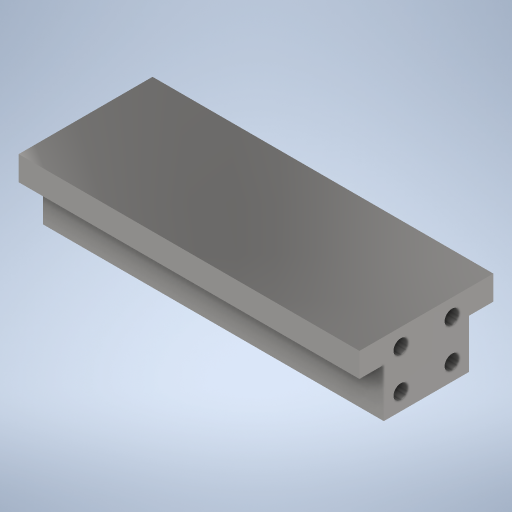
# Autodesk Inventor part: Fuhrung
Saved by Autodesk Inventor 2023.2 (Build 272271000, 271)
## iProperties
Created: 2023-02-02
Part Number: Fuhrung
Material: Steel, Mild
Document SubType Name: Modeling
Designer: Aditya
Density: 7.85 g/cm^3
Appearance: Semi-Polished
Author: Aditya
Autodesk Inventor part; units mm, degrees
ref_plane "YZ Plane" through (0, 0, 0) normal (1, 0, 0) x (0, 1, 0)
ref_plane "XZ Plane" through (0, 0, 0) normal (0, 1, 0) x (-1, 0, 0)
ref_plane "XY Plane" through (0, 0, 0) normal (0, 0, 1) x (1, 0, 0)
sketch "Sketch1" plane through (0, 0, 0) normal (1, 0, 0) x (0, 1, 0)
  line L0 (30, 0) -> (30, -55)
  line L1 (30, -55) -> (20, -55)
  line L2 (20, -55) -> (20, -45)
  line L3 (20, -45) -> (0, -45)
  line L4 (0, -45) -> (0, -10)
  line L5 (0, -10) -> (20, -10)
  line L6 (20, -10) -> (20, 0)
  line L7 (20, 0) -> (30, 0)
  point P0 (0, 0)
  dimension "d0" = 55
  dimension "d1" = 10
  dimension "d2" = 10
  dimension "d3" = 20
  dimension "d4" = 35
  dimension "d5" = 20
  dimension "d6" = 10
  dimension "d7" = 30
  dimension "d8" = 0
  constraints: 16 end point, 4 perpendicular, 2 point on line, 1 vertical
  measures "d0" distance of L0.start L0.end
  measures "d1" distance of L0.end L1.end
  measures "d2" distance of L1.end L2.end
  measures "d3" distance of L2.end L3.end
  measures "d4" distance of L3.end L4.end
  measures "d5" distance of L4.end L5.end
  measures "d6" distance of L5.end L6.end
  measures "d7" distance from line of point (0, 0) L0
  measures "d8" distance from line of point (0, 0) L7
extrude "Extrusion1" add sketch "Sketch1" against normal blind 140
sketch "Sketch3" plane through (0, 0, 0) normal (1, 0, 0) x (0, 0, -1)
  line L0 (55, 30) -> (0, 30) projected
  line L1 (10, 20) -> (10, 0) projected
  line L2 (45, 0) -> (45, 20) projected
  line L3 (10, 0) -> (45, 0) projected
  point P0 (0, 0)
  point P1 (17, 23)
  point P2 (38, 23)
  point P3 (17, 7)
  point P4 (38, 7)
  dimension "d26" = 7
  dimension "d27" = 7
  dimension "d28" = 7
  dimension "d29" = 7
  dimension "d30" = 7
  dimension "d31" = 7
  dimension "d32" = 7
  dimension "d33" = 7
  measures "d26" distance from line of L0 point (17, 23)
  measures "d27" distance from line of L1 point (17, 23)
  measures "d28" distance from line of L0 point (38, 23)
  measures "d29" distance from line of L2 point (38, 23)
  measures "d30" distance from line of L3 point (17, 7)
  measures "d31" distance from line of L3 point (38, 7)
  measures "d32" distance from line of L2 point (38, 7)
  measures "d33" distance from line of L1 point (17, 7)
hole "Hole2" at (0, 23, -17) at (0, 23, -38) at (0, 7, -38) at (0, 7, -17) direction (-1, 0, 0) diameter 4.917 depth 20 tip angle 118 counterbore diameter 6 counterbore depth 15 thread size "M6x1" class "6H" standard "ISO Metric profile"
sketch "Sketch4" plane through (-140, 0, 0) normal (-1, 0, 0) x (0, 0, 1)
  line L0 (-45, 0) -> (-10, 0) projected
  line L1 (-45, 20) -> (-45, 0) projected
  line L2 (-10, 0) -> (-10, 20) projected
  point P0 (0, 0)
  point P1 (-38, 23)
  point P2 (-17, 23)
  point P3 (-27.6865, 8)
  dimension "d41" = 8
  dimension "d42" = 23
  dimension "d43" = 23
  dimension "d44" = 7
  dimension "d45" = 7
  measures "d41" distance from line of L0 point (-27.686, 8)
  measures "d42" distance from line of L0 point (-38, 23)
  measures "d43" distance from line of L0 point (-17, 23)
  measures "d44" distance from line of L1 point (-38, 23)
  measures "d45" distance from line of L2 point (-17, 23)
hole "Hole3" at (-140, 8, -27.6865) at (-140, 23, -38) at (-140, 23, -17) direction (1, 0, 0) diameter 4.917 depth 20 tip angle 118 counterbore diameter 6 counterbore depth 15 thread size "M6x1" class "6H" standard "ISO Metric profile"
sketch "Sketch5" plane through (0, 0, -45) normal (0, -1, 0) x (1, 0, 0)
  line L0 (0, 35) -> (0, 0) projected
  line L1 (0, 45) -> (-140, 45) projected
  line L2 (0, -10) -> (-140, -10) projected
  point P0 (-115, 30)
  point P1 (-70, 30)
  point P2 (-25, 30)
  point P3 (-115, 5)
  point P4 (-70, 5)
  point P5 (-25, 5)
  dimension "d53" = 25
  dimension "d61" = 25
  dimension "d62" = 15
  dimension "d63" = 15
  dimension "d64" = 15
  dimension "d65" = 15
  dimension "d66" = 15
  dimension "d67" = 15
  dimension "d68" = 45
  dimension "d69" = 45
  dimension "d70" = 45
  dimension "d71" = 45
  measures "d53" distance from line of L0 point (-25, 30)
  measures "d61" distance from line of L0 point (-25, 5)
  measures "d62" distance from line of point (-25, 30) L1
  measures "d63" distance from line of L1 point (-70, 30)
  measures "d64" distance from line of L1 point (-115, 30)
  measures "d65" distance from line of L2 point (-25, 5)
  measures "d66" distance from line of L2 point (-70, 5)
  measures "d67" distance from line of L2 point (-115, 5)
  measures "d68" distance of point (-25, 30) point (-70, 30)
  measures "d69" distance of point (-25, 5) point (-70, 5)
  measures "d70" distance of point (-70, 5) point (-115, 5)
  measures "d71" distance of point (-70, 30) point (-115, 30)
hole "Hole4" at (-115, 0, -15) at (-70, 0, -15) at (-115, 0, -40) at (-70, 0, -40) at (-25, 0, -40) at (-25, 0, -15) direction (0, 1, 0) diameter 5.134 depth 16.2 tip angle 118 thread size "M6x0.8" class "6H" standard "ISO Metric profile"
body "Solid1"
